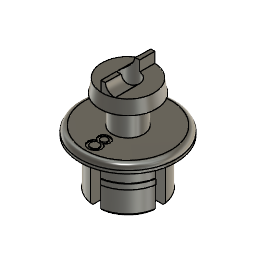
закрутка 8 шлиц v11 (Autodesk Fusion 360 design; units mm, degrees)
Autodesk Fusion 360 part; units mm, degrees
note: some values were not read from the file. Chosen so that the rebuilt part matches the saved one: a direction; the layout of a text. Set by a fixed rule: which sketch regions a step uses.
sketch "Sketch1" plane through (0, 0, 0) normal (0, 1, 0) x (1, 0, 0)
  line L0 (4.2, -37.4) -> (10, -37.4)
  line L1 (10, -37.4) -> (10.8, -32.4)
  line L2 (10.8, -32.4) -> (6, -31)
  line L3 (6, -31) -> (6, -21.6)
  line L4 (6, -21.6) -> (16.5, -21.6)
  line L5 (18.5, -19.6) -> (18.5, -18.5)
  line L6 (18.5, -18.5) -> (13.75, -18.5)
  line L7 (13.75, -18.5) -> (13.75, -18)
  line L8 (13.75, -18) -> (12.59, -18)
  line L9 (12.59, -18) -> (12.59, -15)
  line L10 (12.59, -15) -> (12.6, -15)
  line L11 (12.6, -15) -> (12.6, -1)
  line L12 (11.6, 0) -> (6.2, 0)
  line L13 (4.2, -37.4) -> (4.2, -14)
  line L14 (5.2, -1) -> (5.2, -13)
  line L15 (6.2, 0) -> (5.2, -1)
  line L16 (5.2, -13) -> (4.2, -14)
  arc A0 (16.5, -21.6) -> (18.5, -19.6) centre (16.5, -19.6) ccw
  line L17 (11.6, 0) -> (12.6, -1)
  point P0 (18.5, -21.6)
  dimension "d3" = 10.8
  dimension "d9" = 3
  dimension "d10" = 0.5
  dimension "d11" = 3.1
  dimension "d12" = 10.8
  dimension "d13" = 9.4
  dimension "d16" = 4.2
  dimension "d17" = 6.2
  dimension "d18" = 5.2
  dimension "d19" = 1
  dimension "d20" = 1
  dimension "d21" = 13
  dimension "d22" = 10
  dimension "d24" = 13.75
  dimension "d25" = 18.5
  dimension "d26" = 6
  dimension "d27" = 12.59
  dimension "d28" = 2
  dimension "d29" = 37.4
  dimension "d79" = 1
  dimension "d81" = 1
  dimension "d82" = 15
  dimension "d83" = 12.6
  constraint perpendicular L0 L3
  constraint perpendicular L3 L4
  constraint perpendicular L0 L5
  constraint perpendicular L5 L6
  constraint perpendicular L6 L7
  constraint perpendicular L7 L8
  constraint perpendicular L8 L9
  constraint perpendicular L7 L10
  constraint perpendicular L10 L11
  constraint horizontal L12
  constraint perpendicular L12 L13
  constraint perpendicular L12 L14
  constraint coincident P0 L4
  constraint coincident P0 L5
  constraint tangent L4 A0
  constraint tangent L5 A0
  constraint vertical L3
  measures "d3" horizontal distance of origin L1.end
  measures "d9" distance of L8.end L9.end
  measures "d10" distance of L6.end L7.end
  measures "d11" distance of P0 L5.end
  measures "d12" distance of L1.end L4
  measures "d13" distance of L2.end L4
  measures "d16" distance of origin L13
  measures "d17" distance of origin L12.end
  measures "d18" horizontal distance of origin L14.start
  measures "d19" vertical distance of L14.end L13.end
  measures "d20" vertical distance of L12.end L14.start
  measures "d21" vertical distance of origin L14.end
  measures "d22" horizontal distance of origin L0.end
  measures "d24" horizontal distance of origin L7.end
  measures "d25" horizontal distance of origin P0
  measures "d26" distance of origin L3
  measures "d27" horizontal distance of origin L9.end
  measures "d28" radius of A0
  measures "d29" vertical distance of origin L0.start
  measures "d79" horizontal distance of L12.start L11.end
  measures "d81" vertical distance of L12.start L11.end
  measures "d82" vertical distance of origin L10.end
  measures "d83" horizontal distance of origin L11.end
revolve "Revolve2" add sketch "Sketch1" angle 360 about axis through (0, 0, 1.75) along (0, 0, 1) makes body 1
sketch "Sketch2" plane through (0, 0, 0) normal (0, 0, -1) x (1, 0, 0)
  circle A0 centre (0, 0) radius 8.2
  circle A1 centre (0, 0) radius 12.6
  line L0 (14, -2) -> (-14, -2)
  line L1 (-14, -2) -> (-14, 2)
  line L2 (-14, 2) -> (14, 2)
  line L3 (14, 2) -> (14, -2)
  line L4 (14, -2) -> (-14, 2) construction
  line L5 (-14, -2) -> (14, 2) construction
  line L6 (2, -15) -> (-2, -15)
  line L7 (-2, -15) -> (-2, 15)
  line L8 (-2, 15) -> (2, 15)
  line L9 (2, 15) -> (2, -15)
  line L10 (2, -15) -> (-2, 15) construction
  line L11 (-2, -15) -> (2, 15) construction
  dimension "d31" = 4
  dimension "d32" = 4
  constraint horizontal L0
  constraint perpendicular L0 L1
  constraint parallel L0 L2
  constraint parallel L1 L3
  constraint coincident L4 A0.centre
  constraint coincident L5 A0.centre
  constraint coincident A0.centre A1.centre
  constraint horizontal L6
  constraint perpendicular L6 L7
  constraint parallel L6 L8
  constraint parallel L7 L9
  constraint coincident L10 A0.centre
  constraint coincident L11 A0.centre
  measures "d31" distance of L7.end L8.end
  measures "d32" distance of L0.start L2.end
extrude "Extrude3" cut sketch "Sketch2" against normal blind 17 contours A0 L0 L2 L9 | A0 A1 L0 L2 | A0 L2 L7 L9 | A0 A1 L7 L9 | A0 A1 L7 L9 | A0 L0 L7 L9 | A0 L0 L2 L7 | A0 A1 L0 L2 bodies 1
fillet "Fillet1" radius 2 2 edges at (8.0617, 2, 17) (8.0617, -2, 17) on bodies 1
fillet "Fillet1" radius 2 6 edges at (2, -8.0617, 17) (-2, -8.0617, 17) (-2, 8.0617, 17) (2, 8.0617, 17) (-8.0617, 2, 17) (-8.0617, -2, 17) on bodies 1
sketch "Sketch4" plane through (0, 0, 37.4) normal (0, 0, 1) x (-1, 0, 0)
  circle A0 centre (0, 0) radius 10
  circle A1 centre (0, 0) radius 4.2
  circle A2 centre (0, 0) radius 4.2 construction
  circle A3 centre (0, 0) radius 10 construction
  line L0 (-0.3267, -13) -> (4.1733, -13)
  line L1 (4.1733, -13) -> (4.1733, -0.4732)
  line L2 (4.1733, -0.4732) -> (-0.3267, -0.4732)
  line L3 (-0.3267, -0.4732) -> (-0.3267, -13)
  dimension "d106" = 4.5
  constraint horizontal L0
  constraint vertical L1
  constraint horizontal L2
  constraint vertical L3
  constraint coincident A2 L1.end
  measures "d106" distance of L1.end L2.end
extrude "Extrude4" add sketch "Sketch4" along normal blind 4 contours A0 A1 L1 L3 picked at (2.891, -7.5182) bodies 1
ref_plane "WorkPlane1" through (0.3267, 9.9947, 41.4) normal (0.032674, 0.999466, 0) x (-0.999466, 0.032674, 0)
sketch "Sketch5" plane through (0.3267, 9.9947, 0) normal (0.032674, 0.999466, 0) x (0.999466, -0.032674, 0)
  line L0 (-4.468, -41.4) -> (0, -41.4)
  line L1 (-4.468, -37.4) -> (-4.468, -41.4)
  arc A0 (-1.5, -41.4) -> (-4.468, -37.4) centre (-6.3943, -41.9305) ccw
  point P0 (-4.468, -41.4)
  dimension "d105" = 1.5
  constraint coincident L1.start A0.end
  constraint coincident L0 A0.start
  measures "d105" distance of L0.end A0.start
extrude "Extrude5" cut sketch "Sketch5" against normal blind 10 bodies 1
pattern_circular "C-Pattern1" count 2 over 360 about axis through (0, 0, 1.75) along (0, 0, 1) of "Extrude4", "Extrude5"
ref_plane "WorkPlane2" through (-8.0667, -2, 8.5) normal (0, 1, 0) x (-1, 0, 0)
sketch "Sketch6" plane through (0, -2, 0) normal (0, 1, 0) x (1, 0, 0)
  line L0 (-12.5, -11.2) -> (-12.8, -11.2)
  line L1 (-12.8, -11.2) -> (-12.8, -9.2)
  line L2 (-12.8, -9.2) -> (-12.5, -9.2)
  line L3 (-12.5, -9.2) -> (-12.5, -11.2)
  point P0 (-12.4403, 0)
  dimension "d56" = 9.2
  dimension "d57" = 2
  dimension "d58" = 0.3
  constraint horizontal L0
  constraint vertical L1
  constraint horizontal L2
  constraint vertical L3
  measures "d56" vertical distance of L2.end P0
  measures "d57" distance of L0.end L1.end
  measures "d58" distance of L0.start L0.end
revolve "Revolve3" add sketch "Sketch6" angle 70 about axis through (0, 0, 1.75) along (0, 0, 1) separate body makes body 2
ref_plane "WorkPlane5" through (-2, 12.4403, 15) normal (0.707107, -0.707107, 0) x (0.707107, 0.707107, 0)
ref_plane "WorkPlane7" through (-3.8383, 3.5082, 6.3297) normal (0.738138, -0.67465, 0) x (-0.67465, -0.738138, 0)
sketch "Sketch9" plane through (-3.8383, 3.5082, 0) normal (0.738138, -0.67465, 0) x (-0.67465, -0.738138, 0)
  line L0 (0.9989, -8.9103) -> (-1.0011, -8.9103)
  line L1 (-1.0011, -8.9103) -> (-1.0011, -1.2837)
  line L2 (-1.0011, -1.2837) -> (0.9989, -1.2837)
  line L3 (0.9989, -1.2837) -> (0.9989, -8.9103)
  line L4 (0.9989, -8.9103) -> (-1.0011, -1.2837) construction
  line L5 (-1.0011, -8.9103) -> (0.9989, -1.2837) construction
  point P0 (-0.0011, -5.097)
  dimension "d85" = 2
  constraint horizontal L0
  constraint perpendicular L0 L1
  constraint parallel L0 L2
  constraint parallel L1 L3
  constraint coincident L4 P0
  constraint coincident L5 P0
  measures "d85" distance of L1.end L2.end
extrude "Extrude6" add sketch "Sketch9" along normal blind 2.1 separate body makes body 3
chamfer "Chamfer1" distance 1 angle 45 4 edges at (-1.6129, 2.8303, 5.097) (-2.9622, 1.3541, 5.097) (-2.2875, 2.0922, 1.2837) (-2.2875, 2.0922, 8.9103) on bodies 3
pattern_circular "C-Pattern3" count 2 over 360 about axis through (0, 0, 1.75) along (0, 0, 1) of bodies 3 makes body 4
ref_plane "WorkPlane8" through (0, 0, 21.6) normal (0, 0, 1) x (1, 0, 0)
sketch "Sketch11" plane through (0, 0, 21.6) normal (0, 0, 1) x (1, 0, 0)
  line L0 (-2.8755, -13.6149) -> (-2.861, -13.6146) construction
  line L1 (-2.861, -13.6146) -> (-3.0407, -5.1804) construction
  line L2 (-3.0407, -5.1804) -> (-3.0552, -5.1807) construction
  line L3 (-3.0552, -5.1807) -> (-2.8755, -13.6149) construction
  dimension "d92" = 8
  text T0 "8" font "Arial" height 8 align left top in box 0.0145 x 8.4362 at (-2.8755, -13.6149) x (0.999773, 0.021298) y (-0.021298, 0.999773) spacing 1 by line height
delete_body "RemoveBody1" bodies 2
extrude "Extrude8" cut sketch "Sketch11" against normal blind 0.4 text T0 bodies 1
sketch "Sketch13" plane through (0, 2, 0) normal (0, -1, 0) x (1, 0, 0)
  line L0 (-3.6932, 15) -> (-12.4301, 15)
  line L1 (-12.4301, 15) -> (-12.4403, 15)
  line L2 (-12.4403, 15) -> (-12.4403, 1)
  spline S0 degree 2 poles (-11.4263, 0) (-11.9123, 0.4788) (-12.4403, 1) knots 0 0 0 0.142413 0.142413 0.142413 weights 1 1.000879 1
  line L3 (-11.4263, 0) -> (-5.8686, 0)
  spline S1 degree 2 poles (-4.8, 1) (-5.2874, 0.5501) (-5.8686, 0) knots 0 0 0 0.14635 0.14635 0.14635 weights 1 1.004422 1
  line L4 (-4.8, 1) -> (-4.8, 13)
  spline S2 degree 2 poles (-3.6932, 14) (-4.1877, 13.5652) (-4.8, 13) knots 0 0 0 0.149164 0.149164 0.149164 weights 1 1.007004 1
  line L5 (-3.6932, 14) -> (-3.6932, 15)
  line L6 (-12.4403, 11.2) -> (-12.7403, 11.2)
  line L7 (-12.7403, 11.2) -> (-12.7403, 9.2)
  line L8 (-12.7403, 9.2) -> (-12.4403, 9.2)
  line L9 (-12.4403, 9.2) -> (-12.4403, 11.2)
  dimension "d99" = 0.3
  dimension "d100" = 2
  dimension "d101" = 9.2
  constraint horizontal L6
  constraint vertical L7
  constraint horizontal L8
  constraint vertical L9
  constraint coincident L2 L6.start
  measures "d99" distance of L6.start L6.end
  measures "d100" distance of L6.end L7.end
  measures "d101" distance of L3 L8
revolve "Revolve4" add sketch "Sketch13" angle 71 about axis through (0, 0, 1.75) along (0, 0, -1) contours L2 L6 L7 L8 L9 bodies 1
pattern_circular "C-Pattern4" count 2 over 180 about axis through (0, 0, 1.75) along (0, 0, 1) both ways of "Revolve4"
extrude "Extrude7" [suppressed]
named bodies: "Шліц", "Шліц (1)"
